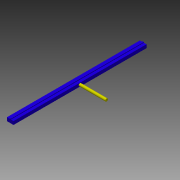
# Autodesk Inventor part: peam
Saved by Autodesk Inventor 2015 (Build 190159000, 159)
## iProperties
Created: 2017-04-05
Part Number: peam
Material: Generic
Document SubType Name: Modeling
Designer: Mohalla
Density: 1 g/cm^3
Appearance: Default
Mass: 1362.83 g
Surface Area: 1751.66 cm^2
Volume: 1362.83 cm^3
Author: Mohalla
Autodesk Inventor part; units mm, degrees
ref_plane "YZ Plane" through (0, 0, 0) normal (1, 0, 0) x (0, 1, 0)
ref_plane "XZ Plane" through (0, 0, 0) normal (0, 1, 0) x (-1, 0, 0)
ref_plane "XY Plane" through (0, 0, 0) normal (0, 0, 1) x (1, 0, 0)
sketch "Sketch1" plane through (0, 0, 0) normal (0, 0, 1) x (1, 0, 0)
  line L0 (0, 5) -> (-5, 5)
  line L1 (-5, 5) -> (-5, 0)
  line L2 (-5, 0) -> (-25, 0)
  line L3 (-25, 0) -> (-25, -25)
  line L4 (-25, -25) -> (25, -25)
  line L5 (25, -25) -> (25, 0)
  line L6 (25, 0) -> (5, 0)
  line L7 (5, 0) -> (5, 5)
  line L8 (5, 5) -> (0, 5)
  point P0 (0, 0)
  dimension "d0" = 5
  dimension "d1" = 5
  dimension "d2" = 5
  dimension "d3" = 5
  dimension "d4" = 50
  dimension "d5" = 25
  dimension "d6" = 25
  dimension "d7" = 20
  dimension "d8" = 5
  constraints: 18 end point, 6 perpendicular, 2 point on line, 1 horizontal
  measures "d0" distance of L6.end L7.end
  measures "d1" distance of L0.end L1.end
  measures "d2" distance of L0.start L0.end
  measures "d3" distance of L7.end L0.start
  measures "d4" distance between parallel lines of L3 L5
  measures "d5" distance of L4.end L5.end
  measures "d6" distance from line of L3 point (0, 0)
  measures "d7" distance of L5.end L6.end
  measures "d8" distance from line of point (0, 0) L0
extrude "Extrusion1" add sketch "Sketch1" along normal mid plane 1000
sketch "Sketch2" plane through (25, -25, 500) normal (1, 0, 0) x (0, 0, -1)
  circle A0 centre (500, 12.5) radius 10
  line L0 (1000, 0) -> (0, 0) projected
  line L1 (0, 0) -> (0, 25) projected
  point P0 (500, 25)
  dimension "d11" = 20
  dimension "d12" = 12.5
  dimension "d13" = 500
  constraints: 1 centre point
  measures "d11" diameter of A0
  measures "d12" distance from line of L0 A0.centre
  measures "d13" distance from line of L1 A0.centre
extrude "Extrusion2" add sketch "Sketch2" along normal blind 200
body "Solid1"
